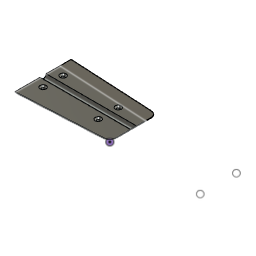
PV panel holder 2 (Autodesk Fusion 360 design; units mm, degrees)
Autodesk Fusion 360 part; units mm, degrees
sketch "Sketch1" plane through (0, 0, 0) normal (0, 0, 1) x (1, 0, 0)
  line L0 (0, 0) -> (-89.8767, -4.7102)
  line L1 (0, 0) -> (90, 0) construction
  line L2 (0, 0) -> (0, 36)
  line L3 (0, 36) -> (-89.8767, 40.7102)
  line L4 (0, 36) -> (90, 36) construction
  line L5 (-89.8767, 40.7102) -> (-89.8767, -4.7102)
  dimension "d1" = 177
  dimension "d2" = 90
  dimension "d3" = 36
  dimension "d4" = 177
  dimension "d5" = 90
  constraint horizontal L1
  constraint coincident L0.start L1.start
  constraint perpendicular L1 L2
  constraint horizontal L4
  measures "d1" angle of L0 L1
  measures "d2" distance of L0.start L0.end
  measures "d3" distance of L0.start L2.end
  measures "d4" angle of L3 L4
  measures "d5" distance of L2.end L3.end
extrude "Extrude1" add sketch "Sketch1" along normal blind 6 draft 45
fillet "Fillet1" radius 10 2 edges at (3, -2.8469, 3) (3, 38.8469, 3)
sketch "Sketch2" plane through (0, 0, 0) normal (0, 0, -1) x (1, 0, 0)
  ellipse E0 centre (-14.1421, -22.5796) end of major axis (-1.7883, -34.3029) minor radius 10 (-6.701, -36.3512) -> (0, -29.2898) ccw
  line L0 (0, -29.2898) -> (0, -6.7102)
  ellipse E1 centre (-14.1421, -13.4204) end of major axis (-1.7883, -1.6971) minor radius 10 (0, -6.7102) -> (-6.701, 0.3512) ccw
  line L1 (-6.701, 0.3512) -> (-89.8767, 4.7102)
  line L2 (-89.8767, 4.7102) -> (-89.8767, -40.7102)
  line L3 (-89.8767, -40.7102) -> (-6.701, -36.3512)
  line L4 (-89.8767, 4.7102) -> (-89.8767, -18) construction
  line L5 (-89.8767, -18) -> (-45.8767, -18) construction
  line L6 (-6.8767, -33.25) -> (-84.8767, -33.25)
  line L7 (-84.8767, -33.25) -> (-84.8767, -2.75)
  line L8 (-84.8767, -2.75) -> (-6.8767, -2.75)
  line L9 (-6.8767, -2.75) -> (-6.8767, -33.25)
  line L10 (-6.8767, -33.25) -> (-84.8767, -2.75) construction
  line L11 (-84.8767, -33.25) -> (-6.8767, -2.75) construction
  point P0 (-45.8767, -18)
  dimension "d10" = 22.7102
  dimension "d11" = 44
  dimension "d12" = 78
  dimension "d13" = 30.5
  constraint coincident L1.end L2.start
  constraint midpoint L2 L4.end
  constraint perpendicular L4 L5
  constraint horizontal L6
  constraint perpendicular L6 L7
  constraint parallel L6 L8
  constraint parallel L7 L9
  constraint coincident L10 P0
  constraint coincident L11 P0
  constraint coincident P0 L5.end
  measures "d10" distance of L1.end L4.end
  measures "d11" distance of L4.end P0
  measures "d12" distance of L7.end L8.end
  measures "d13" distance of L6.end L7.end
extrude "Extrude2" cut sketch "Sketch2" against normal blind 1.5 contours L6 L7 L8 L9
sketch "Sketch3" plane through (0, 0, 0) normal (0, 0, -1) x (1, 0, 0)
  line L0 (-84.8767, -33.25) -> (-84.8767, -2.75)
  line L1 (-84.8767, -2.75) -> (-6.8767, -2.75)
  line L2 (-6.8767, -2.75) -> (-6.8767, -33.25)
  line L3 (-6.8767, -33.25) -> (-84.8767, -33.25)
  ellipse E0 centre (-14.1421, -22.5796) end of major axis (-1.7883, -34.3029) minor radius 10 (-6.701, -36.3512) -> (0, -29.2898) ccw
  line L4 (0, -29.2898) -> (0, -6.7102)
  ellipse E1 centre (-14.1421, -13.4204) end of major axis (-1.7883, -1.6971) minor radius 10 (0, -6.7102) -> (-6.701, 0.3512) ccw
  line L5 (-6.701, 0.3512) -> (-89.8767, 4.7102)
  line L6 (-89.8767, 4.7102) -> (-89.8767, -40.7102)
  line L7 (-89.8767, -40.7102) -> (-6.701, -36.3512)
sketch "Sketch4" plane through (0, 0, 0) normal (0, 0, -1) x (1, 0, 0)
  line L0 (-85, -15) -> (-85, 16.158)
  line L1 (-85, 16.158) -> (-101.3363, 16.158)
  line L2 (-101.3363, 16.158) -> (-101.3363, -48.0286)
  line L3 (-101.3363, -48.0286) -> (-85, -48.0286)
  line L4 (-85, -48.0286) -> (-85, -15)
  constraint vertical L0
  constraint perpendicular L0 L1
  constraint perpendicular L1 L2
  constraint perpendicular L2 L3
  constraint perpendicular L3 L4
extrude "Extrude3" cut sketch "Sketch4" against normal blind 15
sketch "Sketch5" plane through (-85, 0, 0) normal (-1, 0, 0) x (0, -1, 0)
  line L0 (4.4547, 0) -> (10.4629, 6)
  line L1 (10.4629, 6) -> (-46.4629, 6)
  line L2 (-46.4629, 6) -> (-40.4547, 0)
  line L3 (-40.4547, 0) -> (4.4547, 0)
  line L4 (-46.4629, 6) -> (-18, 6)
  line L5 (10.4629, 6) -> (-18, 6)
  circle A0 centre (-18, 6) radius 3
  dimension "d18" = 28.4629
  dimension "d19" = 6
  constraint coincident L1.end L2.start
  constraint midpoint L1 L4.end
  constraint parallel L4 L5
  constraint coincident L4.end L5.end
  measures "d18" distance of L4.end L0.end
  measures "d19" diameter of A0
extrude "Extrude4" cut sketch "Sketch5" against normal blind 100 contours L1 L4 L5 A0 picked at (-19.9888, 5.851)
chamfer "Chamfer1" distance 0.5 angle 45 10 edges at (-42.8505, -8.2539, 6) (6, 8.0082, 6) (4.2117, -3.9967, 6) (3, 18, 3) (6, 27.9918, 6) (-42.8505, 44.2539, 6) (4.2117, 39.9967, 6) (-85, 33.7314, 6) (-85, 18, 3) (-85, 2.2686, 6)
chamfer "Chamfer2" distance 0.5 angle 45 10 edges at (-1.7883, 34.3029, 0) (-45.8505, 38.4029, 0) (-45.8505, -2.4029, 0) (-1.7883, 1.6971, 0) (0, 18, 0) (-85, -7.2084, 2.75) (-85, 43.2084, 2.75) (-45.8767, 33.25, 0) (-6.8767, 18, 0) (-45.8767, 2.75, 0)
sketch "Sketch6" plane through (0, 0, 6) normal (0, 0, 1) x (-1, 0, 0)
  spline S0 degree 3 poles (-5.2935, -15) (-5.3627, -14.9531) (-5.4315, -14.9058) (-5.5, -14.8582) knots 0 0 0 0 0.025071 0.025071 0.025071 0.025071
  line L0 (-5.2935, -15) -> (84.5, -15)
  line L1 (84.5, -15) -> (84.5, 9.936)
  line L2 (84.5, 9.936) -> (1.0622, 5.5632)
  line L3 (0.7272, 5.5457) -> (1.0622, 5.5632)
  spline S1 degree 3 poles (-5.5, -1.0164) (-5.5, -0.8241) (-5.4943, -0.6349) (-5.4197, 0.5909) (-5.1793, 1.5237) (-4.5302, 2.8177) (-4.2188, 3.2629) (-3.849, 3.6526) (-3.4792, 4.0422) (-3.051, 4.3765) (-1.7926, 5.0924) (-0.8738, 5.3813) (0.3465, 5.52) (0.5351, 5.5356) (0.7272, 5.5457) knots -0.508354 -0.508354 -0.508354 -0.508354 -0.45799 -0.45799 -0.17615 -0.17615 0 0 0 0.17615 0.17615 0.45799 0.45799 0.508354 0.508354 0.508354 0.508354
  line L4 (-5.5, -1.3519) -> (-5.5, -1.0164)
  line L5 (-5.5, -1.3519) -> (-5.5, -14.8582)
  line L6 (82, -17.9581) -> (47, -17.9581) construction
  line L7 (74.5, -7.9581) -> (19.5, -7.9581) construction
  line L8 (19.5, -7.9581) -> (19.5, -27.9581) construction
  line L9 (19.5, -27.9581) -> (74.5, -27.9581) construction
  line L10 (74.5, -27.9581) -> (74.5, -7.9581) construction
  line L11 (74.5, -7.9581) -> (19.5, -27.9581) construction
  line L12 (19.5, -7.9581) -> (74.5, -27.9581) construction
  point P0 (47, -17.9581)
  dimension "d24" = 35
  dimension "d25" = 55
  dimension "d26" = 20
  constraint perpendicular L1 L6
  constraint horizontal L7
  constraint perpendicular L7 L8
  constraint parallel L7 L9
  constraint parallel L8 L10
  constraint coincident L11 P0
  constraint coincident L12 P0
  constraint coincident P0 L6.end
  measures "d24" distance of L6.start P0
  measures "d25" distance of L8.end L9.end
  measures "d26" distance of L7.end L8.end
hole "Hole1" at (-19.5, 27.9581, 6) at (-19.5, 7.9581, 6) at (-74.5, 27.9581, 6) at (-74.5, 7.9581, 6) direction (0, 0, -1) diameter 3 depth 10 tip angle 118 countersink diameter 6 countersink angle 90
